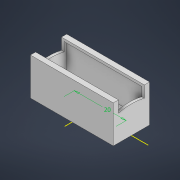
# Autodesk Inventor part: Test_Switch_Housing
Saved by Autodesk Inventor 2022 (Build 260153000, 153)
## iProperties
Created: 2024-05-10
Part Number: Test_Switch_Housing
Material: Generic
Document SubType Name: Modeling
Designer: jo_ki
Density: 1 g/cm^3
Appearance: Default
Author: jo_ki
Autodesk Inventor part; units mm, degrees
ref_plane "YZ Plane" through (0, 0, 0) normal (1, 0, 0) x (0, 1, 0)
ref_plane "XY Plane" through (0, 0, 0) normal (0, 0, 1) x (1, 0, 0)
sketch "Sketch5" plane through (0, 0, 0) normal (1, 0, 0) x (0, 1, 0)
  line L0 (5, 7) -> (-6, 7)
  line L1 (-6, 7) -> (-6, -5)
  line L2 (-6, -5) -> (5, -5)
  line L3 (5, -5) -> (5, 7)
  line L4 (-6, -5) -> (5, -5)
  line L5 (5, -5) -> (5, -7)
  line L6 (5, -7) -> (-6, -7)
  line L7 (-6, -7) -> (-6, -5)
  line L8 (5, 7) -> (-6, 7)
  line L9 (-6, 7) -> (-6, 5)
  line L10 (-6, 5) -> (5, 5)
  line L11 (5, 5) -> (5, 7)
  line L12 (-51.3319, 0) -> (14.3886, 0) projected
  line L13 (0, -30.178) -> (0, 30.178) projected
  circle A0 centre (-20.3875, 0) radius 16
  circle A1 centre (-20.3875, 0) radius 21.5557
  line L14 (4, 6) -> (-4.4815, 6)
  line L15 (-4.4815, 6) -> (-4.4815, -6)
  line L16 (-4.4815, -6) -> (4, -6)
  line L17 (4, -6) -> (4, 6)
  circle A2 centre (-20.3875, 0) radius 17
  line L18 (-4.4815, -6) -> (-7.3875, -6)
  line L19 (-7.3875, -6) -> (-7.3875, 6)
  line L20 (-7.3875, 6) -> (-4.4815, 6)
  line L21 (-4.4815, 6) -> (-4.4815, -6)
  line L22 (-6, -7) -> (-9.3875, -7)
  line L23 (-9.3875, -7) -> (-9.3875, 7)
  line L24 (-9.3875, 7) -> (-6, 7)
  line L25 (-6, 7) -> (-6, -7)
  point P0 (0, 0)
  point P1 (0, 7)
  point P2 (-6, 7)
  point P3 (-6, -7)
  point P4 (5, -5)
  point P5 (0.5803, -5)
  point P6 (0.5803, 5)
  point P7 (4, -5)
  point P8 (4, 5)
  point P9 (-4.4815, -6)
  point P10 (-6, 7)
  point P11 (-6, -7)
  point P12 (-4.4815, -6)
  point P13 (-4.4815, 6)
  dimension "d14" = 32
  dimension "d25" = 1
  dimension "d15" = 12
  dimension "d16" = 2
  dimension "d17" = 2
  dimension "d18" = 6
  dimension "d19" = 5
  dimension "d20" = 1
  dimension "d22" = 1
  dimension "d23" = 1
  dimension "d31" = 2
  dimension "d32" = 5
  constraints: 48 end point, 12 parallel, 6 horizontal, 6 perpendicular, 5 point on line, 2 coincident, 2 collinear, 10 other
  measures "d15" distance between parallel lines of L2 L0
  measures "d16" distance between parallel lines of L0 L10
  measures "d17" distance between parallel lines of L6 L2
  measures "d18" distance between parallel lines of L13 L1
  measures "d19" distance between parallel lines of L13 L3
  measures "d20" distance between parallel lines of L11 L17
  measures "d22" distance between parallel lines of L14 L0
  measures "d23" distance between parallel lines of L6 L16
  measures "d31" distance between parallel lines of L19 L23
extrude "Extrusion4" add sketch "Sketch5" along normal mid plane 32 contours L3 L10 L17 L14 A1 L0 | L13 L14 A2 L0 | A1 L14 L13 | A2 L20 A0 L0 | L14 A1 L10 L13 | L13 L10 A2 L14 | L14 L17 L10 A1 | A0 L20 L1 | L1 L20 L19 L12 L23 L24 | A2 L10 L15 | L15 L10 A0 L20 | L13 L12 A2 L10 | L10 A1 L12 L13 | A1 L16 L17 L2 L5 L6 | L6 A2 L16 L13 | L13 L16 A1 | L20 A0 L10 L1 | L1 L12 L19 L20 | L15 A0 L10 | L10 A2 L12 A0 L15 | L6 A0 L18 A2 | L13 L2 A2 L12 | L12 A1 L2 L13 | L16 A2 L2 L13 | L13 L2 A1 L16 | A1 L2 L17 L16 | L10 A0 L15 L12 L1 | L12 L19 L18 L7 L22 L23 | L7 L18 A0 | A0 L12 L15 | A2 L2 L15 A0 L12 | L18 A0 L2 L15 | L15 L2 A2 | L12 L15 A0 L2 L1 | L1 L7 L18 L19 L12 | L7 L2 A0 L18 | A0 L15 L12 | L2 A0 L15
extrude "Extrusion5" cut sketch "Sketch5" along normal mid plane 30 contours L14 A1 L10 L13 | L13 L10 A2 L14 | L14 L17 L10 A1 | A2 L10 L15 | L15 L10 A0 L20 | L13 L12 A2 L10 | L10 A1 L12 L13 | L20 A0 L10 L1 | L1 L12 L19 L20 | L15 A0 L10 | L10 A2 L12 A0 L15 | L13 L2 A2 L12 | L12 A1 L2 L13 | L16 A2 L2 L13 | L13 L2 A1 L16 | A1 L2 L17 L16 | L10 A0 L15 L12 L1 | A0 L12 L15 | A2 L2 L15 A0 L12 | L18 A0 L2 L15 | L15 L2 A2 | L12 L15 A0 L2 L1 | L1 L7 L18 L19 L12 | L7 L2 A0 L18 | A0 L15 L12 | L2 A0 L15
ref_plane "Work Plane2" through (16, -9.3875, 7) normal (0, 1, 0) x (-1, 0, 0)
sketch "Sketch9" plane through (16, -9.3875, 7) normal (0, 1, 0) x (-1, 0, 0)
  line L0 (38.4, -7) -> (-6.4, -7) projected
  line L1 (16, -16.8) -> (16, 2.8) projected
  point P0 (16, -7)
  point P1 (6, -7)
  point P2 (16, -7)
  point P3 (26, -7)
  dimension "d33" = 20
  constraints: 2 point on line, 1 coincident, 1 symmetric about line
  measures "d33" distance of point (6, -7) point (26, -7)
hole "Hole1" at (10, -9.3875, 0) at (-10, -9.3875, 0) direction (0, 1, 0) diameter 3.5 depth 5
hole "Hole2" at (0, -9.3875, 0) direction (0, 1, 0) diameter 5 depth 1
equation "\"d25\" = d20"
equation "\"d17\" = d16"
equation "\"d22\" = d20"
equation "\"d23\" = d22"
body "Solid2"
